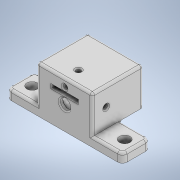
# Autodesk Inventor part: SDM_actuator_mount
Saved by Autodesk Inventor 2021 (Build 250183000, 183)
## iProperties
Created: 2021-06-20
Part Number: SDM_actuator_mount
Material: Generic
Document SubType Name: Modeling
Designer: Charlie
Density: 1 g/cm^3
Appearance: Default
Author: Charlie
Autodesk Inventor part; units mm, degrees
ref_plane "YZ Plane" through (0, 0, 0) normal (1, 0, 0) x (0, 1, 0)
ref_plane "XZ Plane" through (0, 0, 0) normal (0, 1, 0) x (-1, 0, 0)
ref_plane "XY Plane" through (0, 0, 0) normal (0, 0, 1) x (1, 0, 0)
sketch "Sketch1" plane through (0, 0, 0) normal (0, 0, 1) x (1, 0, 0)
  line L0 (-10, 6) -> (10, 6)
  line L1 (10, -6) -> (-10, -6)
  line L2 (-10, -6) -> (-10, 6)
  line L3 (-10, 6) -> (10, -6) construction
  line L4 (10, 6) -> (-10, -6) construction
  line L5 (-6, 1) -> (-6, 3)
  line L6 (-6, 3) -> (6, 3)
  line L7 (6, 3) -> (6, 1)
  line L8 (6, 1) -> (-6, 1)
  circle A0 centre (0, -2) radius 2.25
  line L9 (10, 6) -> (10, -6)
  line L10 (-12, -8) -> (12, -8)
  line L11 (12, -8) -> (12, 8)
  line L12 (12, 8) -> (-12, 8)
  line L13 (-12, 8) -> (-12, -8)
  line L14 (-12, -8) -> (12, 8) construction
  line L15 (12, -8) -> (-12, 8) construction
  circle A1 centre (0, 4.5) radius 1
  point P0 (0, 0)
  point P1 (0, 6)
  dimension "d0" = 20
  dimension "d2" = 2
  dimension "d3" = 12
  dimension "d5" = 4.5
  dimension "d6" = 3
  dimension "d11" = 3
  dimension "d12" = 6
  dimension "d14" = 0
  dimension "d15" = 4
  dimension "d16" = 12
  dimension "d17" = 24
  dimension "d18" = 16
  dimension "d19" = 2
  dimension "d20" = 1.5
  constraints: 32 end point, 5 midpoint, 5 parallel, 2 centre point, 2 horizontal, 2 perpendicular, 1 vertical
  measures "d0" distance of L1.start L1.end
  measures "d2" distance of L6.end L7.end
  measures "d3" distance of L5.end L6.end
  measures "d5" diameter of A0
  measures "d6" distance from line of L8 A0.centre
  measures "d11" vertical distance of L7.end A0.centre
  measures "d12" horizontal distance of L5.start A0.centre
  measures "d14" horizontal distance of point (0, 0) A0.centre
  measures "d15" distance from line of L1 A0.centre
  measures "d16" distance of L4.start L3.end
  measures "d17" distance of L12.end L11.end
  measures "d18" distance of L11.end L10.end
  measures "d19" diameter of A1
  measures "d20" distance from line of A1.centre L6
extrude "Extrusion1" add sketch "Sketch1" along normal blind 2 contours L0 L9 L1 L2 | L13 L12 L11 L10
extrude "Extrusion2" add sketch "Sketch1" against normal blind 20 contours L13 L12 L11 L10
sketch "Sketch2" plane through (-12, -8, 2) normal (0, -1, 0) x (1, 0, 0)
  circle A0 centre (-8, -6) radius 2.3
  line L0 (0, -22) -> (24, -22) construction
  line L1 (12, -22) -> (12, 0) construction
  line L2 (11, 0) -> (13, 0) construction
  line L3 (12, -6) -> (-8, -6) construction
  circle A1 centre (32, -6) radius 2.3
  line L4 (37, -12) -> (-13, -12)
  line L5 (-13, -12) -> (-13, 0)
  line L6 (-13, 0) -> (37, 0)
  line L7 (37, 0) -> (37, -12)
  line L8 (37, -12) -> (-13, 0) construction
  line L9 (-13, -12) -> (37, 0) construction
  point P0 (12, -2)
  point P1 (12, 0)
  dimension "d25" = 4.6
  dimension "d26" = 20
  dimension "d27" = 50
  constraints: 16 end point, 5 midpoint, 2 centre point, 2 horizontal, 2 parallel, 1 coincident, 1 perpendicular
  measures "d25" diameter of A0
  measures "d26" distance of L3.start L3.end
  measures "d27" distance of L5.end L6.end
extrude "Extrusion3" add sketch "Sketch2" along normal blind 4
fillet "Fillet1" radius 2 4 edges at (25, -10, 2) (25, -10, -10) (-25, -10, -10) (-25, -10, 2)
fillet "Fillet1" radius 1 22 edges at (12, 8, -9) (-12, 8, -9) (10, 0, 0) (-10, 0, 0) (18.5, -8, -10) (-18.5, -8, -10) (18.5, -8, 2) (-18.5, -8, 2) (-25, -8, -4) (25, -8, -4) (0, 8, -20) (0, 6, -20) (10, 0, -20) (0, -6, -20) (-10, 0, -20) (12, 0, -20) (-12, 0, -20) (12, 0, 2) (0, 8, 2) (-12, 0, 2) (0, -8, -20) (0, -8, -10)
sketch "Sketch3" plane through (12, -8, -9) normal (1, 0, 0) x (0, 0, -1)
  circle A0 centre (-5, 8) radius 1
  point P0 (-9, 8)
  dimension "d32" = 2
  constraints: 1 centre point
  measures "d32" diameter of A0
extrude "Extrusion4" cut sketch "Sketch3" against normal blind 25
sketch "Sketch4" plane through (-11, 8, -19) normal (0, 1, 0) x (1, 0, 0)
  circle A0 centre (11, -15) radius 1
  circle A1 centre (31, -15) radius 2.3 construction
  circle A2 centre (-9, -15) radius 2.3 construction
  line L0 (31, -15) -> (-9, -15) construction
  point P0 (11, -19)
  dimension "d35" = 2
  constraints: 2 end point, 1 centre point, 1 horizontal, 1 midpoint
  measures "d35" diameter of A0
extrude "Extrusion5" cut sketch "Sketch4" against normal blind 10
chamfer "Chamfer1" distance 0.5 angle 45 6 edges at (-1, 8, -4) (12, 0, -3) (-12, 0, -3) (-1, 4.5, 2) (-2.25, -2, 0) (-2.25, -2, 2)
body "Solid1"
